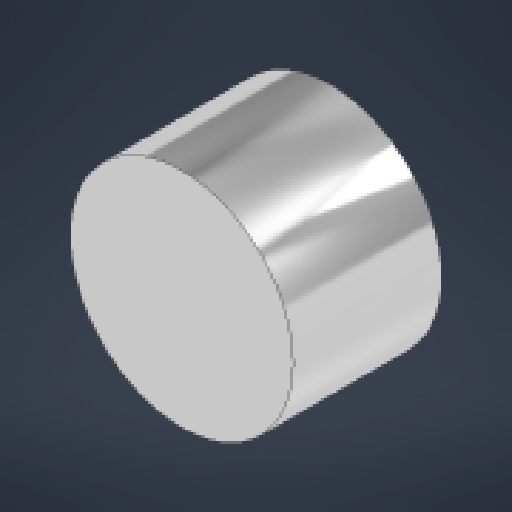
# Autodesk Inventor part: Pogo_Magnet1
Saved by Autodesk Inventor 2026 (Build 300175000, 175)
## iProperties
Created: 2025-04-17
Part Number: Pogo_Magnet1
Material: Nickel-Copper Alloy 400
Document SubType Name: Modeling
Designer: ct_vi
Density: 8.83 g/cm^3
Appearance: Chrome - Polished
Author: ct_vi
Autodesk Inventor part; units mm, degrees
ref_plane "YZ Plane" through (0, 0, 0) normal (1, 0, 0) x (0, 1, 0)
ref_plane "XZ Plane" through (0, 0, 0) normal (0, 1, 0) x (-1, 0, 0)
ref_plane "XY Plane" through (0, 0, 0) normal (0, 0, 1) x (1, 0, 0)
sketch "Sketch1" plane through (0, 0, 0) normal (0, 0, 1) x (1, 0, 0)
  circle A0 centre (5.4, 0) radius 1.5
  point P0 (0, 0)
  dimension "d1" = 3
  constraints: 1 centre point
  measures "d1" diameter of A0
extrude "Extrusion1" add sketch "Sketch1" against normal blind 2
body "Solid1"
